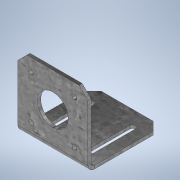
# Autodesk Inventor part: Motor Mount
Saved by Autodesk Inventor 2022 (Build 260153000, 153)
## iProperties
Created: 2021-10-06
Part Number: Motor Mount
Material: Generic
Document SubType Name: Sheet Metal
Designer: nicol
Density: 1 g/cm^3
Sheet Metal Rule: Default
Appearance: Steel Galvanized
Author: nicol
Autodesk Inventor part; units mm, degrees
ref_plane "YZ Plane" through (0, 0, 0) normal (1, 0, 0) x (0, 1, 0)
ref_plane "XZ Plane" through (0, 0, 0) normal (0, 1, 0) x (-1, 0, 0)
ref_plane "XY Plane" through (0, 0, 0) normal (0, 0, 1) x (1, 0, 0)
sketch "Sketch1" plane through (0, 0, 0) normal (0, 0, 1) x (1, 0, 0)
  line L0 (0, 0) -> (50, 0)
  line L1 (50, 0) -> (50, 100)
  line L2 (50, 100) -> (0, 100)
  line L3 (0, 100) -> (0, 0)
  line L4 (0, 51) -> (50, 51)
  line L5 (10, 41) -> (10, 11) construction
  line L6 (7.9, 41) -> (7.9, 11)
  line L7 (12.1, 11) -> (12.1, 41)
  arc A0 (12.1, 41) -> (7.9, 41) centre (10, 41) ccw
  arc A1 (7.9, 11) -> (12.1, 11) centre (10, 11) ccw
  line L8 (40, 41) -> (40, 11) construction
  line L9 (37.9, 41) -> (37.9, 11)
  line L10 (42.1, 11) -> (42.1, 41)
  arc A2 (42.1, 41) -> (37.9, 41) centre (40, 41) ccw
  arc A3 (37.9, 11) -> (42.1, 11) centre (40, 11) ccw
  line L11 (25, 51) -> (25, 0) construction
  line L12 (25, 26) -> (40, 26) construction
  line L13 (25, 26) -> (10, 26) construction
  line L14 (9.5, 91) -> (40.5, 91) construction
  line L15 (40.5, 91) -> (40.5, 60) construction
  line L16 (40.5, 60) -> (9.5, 60) construction
  line L17 (9.5, 60) -> (9.5, 91) construction
  line L18 (0, 100) -> (50, 51) construction
  line L19 (9.5, 91) -> (40.5, 60) construction
  point P0 (25, 75.5)
  point P1 (25, 75.5)
  dimension "d0" = 50
  dimension "d1" = 100
  dimension "d2" = 30
  dimension "d3" = 2.1
  dimension "d4" = 11
  dimension "d5" = 30
  dimension "d6" = 49
  dimension "d7" = 31
  dimension "d8" = 31
  constraints: 44 end point, 8 point on circle, 8 tangent, 7 parallel, 6 midpoint, 4 centre point, 4 horizontal, 3 coincident, 3 perpendicular, 3 point on line, 2 equal length, 1 equal radius, 1 horizontal alignment, 1 vertical
  measures "d0" distance of L0.start L0.end
  measures "d1" distance of L0.end L1.end
  measures "d2" distance of L8.start L8.end
  measures "d3" radius of A0
  measures "d4" distance from line of L0 L8.end
  measures "d5" distance between parallel lines of L5 L8
  measures "d6" distance between parallel lines of L2 L4
  measures "d7" distance of L14.start L14.end
  measures "d8" distance of L14.end L15.end
extrude "Plate1" add sketch "Sketch1" along normal blind 2.286
fold "Fold1" angle 90 bend radius 2.286 thickness 2.286 k factor 0.44 line from (0, 51, 0) to (50, 51, 0) line at bend centre moving side (0, -1, 0) folds toward (0, 0, -1)
hole "Hole1" at (9.5, 91, 0) at (9.5, 60, 0) at (40.5, 91, 0) at (40.5, 60, 0) direction (0, 0, 1) diameter 3.4 end through all clearance for "Socket Head Cap Screw" size "M3" standard "Ansi Metric M Profile"
hole "Hole2" at (25, 75.5, 0) direction (0, 0, 1) diameter 22 end through all
chamfer "Corner Chamfer1" distance 6.35 angle 45 4 edges at (0, 50.1564, -50.7006) (50, 50.1564, -50.7006) (0, 100, 1.143) (50, 100, 1.143)
equation "\"d8\" = d7"
equation "\"d9\" = Thickness"
equation "\"d10\" = BendReliefWidth"
equation "\"d11\" = BendReliefDepth"
equation "\"d12\" = MinimumRemnant"
equation "\"d13\" = TransitionRadius"
equation "\"d15\" = BendRadius"
equation "\"d21\" = Thickness"
equation "\"BendRadius\" = Thickness"
equation "\"BendReliefWidth\" = Thickness"
equation "\"BendReliefDepth\" = 0.5 * Thickness"
equation "\"CornerReliefSize\" = 4 * Thickness"
equation "\"MinimumRemnant\" = 2 * Thickness"
equation "\"TransitionRadius\" = BendRadius"
equation "\"JacobiRadiusSize\" = BendRadius"
equation "\"GapSize\" = Thickness"
equation "\"Thickness\" = 2.286"
body "Solid1"
